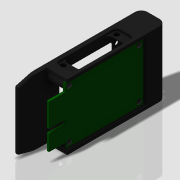
# Autodesk Inventor part: HighSpeedIOShield01
Saved by Autodesk Inventor 2013 (Build 170138000, 138)
## iProperties
Created: 2014-07-14
Part Number: HighSpeedIOShield01
Material: PCB(1)
Document SubType Name: Modeling
Designer: spichelh
Density: 1 g/cm^3
Author: spichelh
Autodesk Inventor part; units mm, degrees
ref_plane "YZ Plane" through (0, 0, 0) normal (1, 0, 0) x (0, 1, 0)
ref_plane "XZ Plane" through (0, 0, 0) normal (0, 1, 0) x (-1, 0, 0)
ref_plane "XY Plane" through (0, 0, 0) normal (0, 0, 1) x (1, 0, 0)
sketch "Sketch1" plane through (0, 0, 0) normal (1, 0, 0) x (0, 1, 0)
  line L0 (0, 0) -> (27.94, 0)
  line L1 (27.94, 0) -> (27.94, 38.1)
  line L2 (13.97, 0) -> (13.97, 11.6982) construction
  circle A0 centre (2, 2) radius 1.25
  circle A1 centre (25.94, 2) radius 1.25
  line L3 (0, 38.1) -> (2.74, 38.1)
  line L4 (2.74, 38.1) -> (2.74, 46)
  line L5 (2.74, 46) -> (10.54, 46)
  line L6 (10.54, 46) -> (10.54, 38.1)
  line L7 (10.54, 38.1) -> (12.54, 38.1)
  line L8 (12.54, 38.1) -> (12.54, 46)
  line L9 (12.54, 46) -> (24.04, 46)
  line L10 (24.04, 46) -> (24.04, 38.1)
  line L11 (24.04, 38.1) -> (27.94, 38.1)
  line L12 (0, 0) -> (0, 38.1)
  circle A2 centre (2, 36.1) radius 1.25
  circle A3 centre (25.94, 36.1) radius 1.25
  point P0 (13.97, 5.8491)
  dimension "d0" = 27.94
  dimension "d5" = 2.5
  dimension "d6" = 2
  dimension "d21" = 7.8
  dimension "d23" = 2
  dimension "d24" = 11.5
  dimension "d27" = 38.1
  dimension "d29" = 3.9
  dimension "d30" = 7.9
  dimension "d31" = 2
  dimension "d32" = 2.5
  dimension "d33" = 2
  dimension "d34" = 2
  constraints: 27 end point, 4 centre point, 3 collinear, 2 midpoint, 2 perpendicular, 2 symmetric about line, 2 vertical, 1 horizontal, 1 parallel, 2 other
  measures "d0" distance of L0.start L0.end
  measures "d5" diameter of A0
  measures "d6" distance from line of L0 A0.centre
  measures "d21" distance between parallel lines of L6 L4
  measures "d23" distance between parallel lines of L6 L8
  measures "d24" distance between parallel lines of L8 L10
  measures "d27" distance of L1.end L0.end
  measures "d29" distance between parallel lines of L10 L1
  measures "d30" distance between parallel lines of L3 L5
  measures "d31" distance from line of L12 A0.centre
  measures "d32" diameter of A2
  measures "d33" distance from line of L12 A2.centre
  measures "d34" distance from line of L3 A2.centre
extrude "Extrusion1" add sketch "Sketch1" along normal blind 1
sketch "Sketch2" plane through (0, 0, 0) normal (-1, 0, 0) x (0, 0, 1)
  circle A0 centre (2, 25.94) radius 1.25 projected
  circle A1 centre (2, 2) radius 1.25 projected
  circle A2 centre (36.1, 25.94) radius 1.25 projected
  circle A3 centre (36.1, 2) radius 1.25 projected
  circle A4 centre (36.1, 2) radius 2
  circle A5 centre (36.1, 25.94) radius 2
  circle A6 centre (2, 25.94) radius 2
  circle A7 centre (2, 2) radius 2
  dimension "d35" = 4
  dimension "d38" = 4
  dimension "d39" = 4
  dimension "d40" = 4
  constraints: 4 centre point, 4 coincident
  measures "d35" diameter of A4
  measures "d38" diameter of A5
  measures "d39" diameter of A6
  measures "d40" diameter of A7
extrude "Extrusion2" add sketch "Sketch2" along normal blind 8
sketch "Sketch3" plane through (-8, 25.94, 2) normal (-1, 0, 0) x (0, 0, 1)
  line L0 (44, -1.9) -> (44, -13.4) projected
  line L1 (44, 4) -> (50, 2.3923)
  line L2 (50, 2.3923) -> (50, -26.3323)
  line L3 (50, -26.3323) -> (45.0725, -27.6526)
  line L4 (45.0725, -27.6526) -> (44, -27.94)
  line L5 (44, -27.94) -> (-4, -27.94)
  line L6 (-4, -27.94) -> (-4, 4)
  line L7 (-4, 4) -> (44, 4)
  line L8 (-2, -25.94) -> (-2, 2) projected
  line L9 (-2, 2) -> (36.1, 2) projected
  line L10 (36.1, -25.94) -> (-2, -25.94) projected
  dimension "d43" = 105
  dimension "d44" = 105
  dimension "d45" = 2
  dimension "d46" = 2
  dimension "d47" = 2
  dimension "d48" = 6
  constraints: 14 end point, 3 perpendicular, 2 point on line, 1 collinear, 1 parallel
  measures "d43" angle of L1 L2
  measures "d44" angle of L3 L2
  measures "d45" distance between parallel lines of L6 L8
  measures "d46" distance between parallel lines of L7 L9
  measures "d47" distance between parallel lines of L5 L10
  measures "d48" distance between parallel lines of L0 L2
extrude "Extrusion3" add sketch "Sketch3" along normal blind 2
sketch "Sketch4" plane through (-8, 25.94, 2) normal (1, 0, 0) x (0, 0, -1)
  line L0 (-44, -27.94) -> (4, -27.94) projected
  line L1 (4, -27.94) -> (4, 4) projected
  line L2 (4, 4) -> (-44, 4) projected
  line L3 (2.5, 2.5) -> (2.5, -26.44)
  line L4 (2.5, -26.44) -> (-36.1, -26.44)
  line L5 (-36.1, 2) -> (-36.1, -1.9) projected
  line L6 (-36.1, 2.5) -> (-36.1, 4)
  line L7 (-36.1, -26.44) -> (-36.1, -27.94)
  line L8 (-36.1, 2.5) -> (2.5, 2.5)
  point P0 (2, -25.94)
  dimension "d51" = 1.5
  dimension "d52" = 1.5
  dimension "d53" = 1.5
  constraints: 10 end point, 2 collinear, 2 perpendicular, 2 point on line
  measures "d51" distance between parallel lines of L3 L1
  measures "d52" distance between parallel lines of L2 L8
  measures "d53" distance between parallel lines of L0 L4
extrude "Extrusion4" add sketch "Sketch4" along normal blind 10
fillet "Fillet1" radius 1 4 edges at (-3, 28.44, -0.5) (-3, -0.5, -0.5) (-9, 28.3323, 52) (-9, -0.3923, 52)
fillet "Fillet2" radius 1 10 edges at (-8, -0.2337, 51.7934) (-8, -1.2955, 48.6294) (-8, 28.1737, 51.7934) (-8, 29.2355, 48.6294) (-8, 13.97, 52) (-10, 13.97, 52) (-10, -0.2337, 51.7934) (-10, -1.2955, 48.6294) (-10, 29.2355, 48.6294) (-10, 28.1737, 51.7934)
thread "Thread1" size "M3x0.5" class "6H" standard "ANSI Metric M Profile" full length
thread "Thread2" size "M3x0.5" class "6H" standard "ANSI Metric M Profile" full length
thread "Thread3" size "M3x0.5" class "6H" standard "ANSI Metric M Profile" full length
thread "Thread4" size "M3x0.5" class "6H" standard "ANSI Metric M Profile" full length
sketch "Sketch6" plane through (2, -2, -2) normal (0, 0, -1) x (-1, 0, 0)
  line L0 (8.5, 30.44) -> (3.5, 30.44)
  line L1 (1.5, 28.44) -> (1.5, 3.5)
  line L2 (3.5, 1.5) -> (8.5, 1.5)
  line L3 (10.5, 3.5) -> (10.5, 28.44)
  arc A0 (3.5, 30.44) -> (1.5, 28.44) centre (3.5, 28.44) ccw
  arc A1 (10.5, 28.44) -> (8.5, 30.44) centre (8.5, 28.44) ccw
  arc A2 (8.5, 1.5) -> (10.5, 3.5) centre (8.5, 3.5) ccw
  arc A3 (1.5, 3.5) -> (3.5, 1.5) centre (3.5, 3.5) ccw
  line L4 (12, 31.94) -> (0, 31.94) projected
  line L5 (12, 31.94) -> (12, 0) projected
  line L6 (12, 0) -> (0, 0) projected
  line L7 (0, 0) -> (0, 31.94) projected
  dimension "d106" = 2
  dimension "d107" = 1.5
  dimension "d108" = 1.5
  dimension "d109" = 1.5
  dimension "d110" = 1.5
  constraints: 8 end point, 8 point on circle, 8 tangent, 4 centre point, 3 equal radius, 2 parallel, 1 horizontal, 1 perpendicular
  measures "d106" radius of A0
  measures "d107" distance between parallel lines of L4 L0
  measures "d108" distance between parallel lines of L3 L5
  measures "d109" distance between parallel lines of L6 L2
  measures "d110" distance between parallel lines of L7 L1
extrude "Extrusion6" cut sketch "Sketch6" against normal blind 0.1 contours A1 L3 A2 L2 A3 L1 A0 L0
sketch "Sketch7" plane through (-10, 25.94, 2) normal (-1, 0, 0) x (0, 0, 1)
  line L0 (40.1363, 4) -> (-4, 4) projected
  line L1 (1.46, -1) -> (32, -1)
  line L2 (34, -3) -> (34, -20.94)
  line L3 (32, -22.94) -> (1.46, -22.94)
  line L4 (-0.54, -20.94) -> (-0.54, -3)
  arc A0 (34, -3) -> (32, -1) centre (32, -3) ccw
  arc A1 (1.46, -1) -> (-0.54, -3) centre (1.46, -3) ccw
  arc A2 (-0.54, -20.94) -> (1.46, -22.94) centre (1.46, -20.94) ccw
  arc A3 (32, -22.94) -> (34, -20.94) centre (32, -20.94) ccw
  line L5 (-4.54, 4) -> (-4.54, -27.94) projected
  line L6 (-4, -27.94) -> (40.1363, -27.94) projected
  line L7 (49, 1.625) -> (49, -25.565) projected
  point P0 (-3.54, 4.54)
  point P1 (-2, -25.94)
  point P2 (34, -22.94)
  point P3 (34, -1)
  point P4 (-0.54, -22.94)
  point P5 (-4, 4)
  dimension "d83" = 2
  dimension "d84" = 5
  dimension "d85" = 4
  dimension "d136" = 5
  dimension "d137" = 15
  constraints: 8 end point, 8 point on circle, 8 tangent, 6 point on line, 4 centre point, 3 equal radius, 2 parallel, 1 horizontal, 1 perpendicular, 1 other
  measures "d83" radius of A0
  measures "d85" distance between parallel lines of L5 L4
  measures "d136" distance between parallel lines of L6 L3
  measures "d137" distance between parallel lines of L7 L2
extrude "Extrusion7" cut sketch "Sketch7" against normal blind 1
sketch "Sketch8" plane through (-10, -2, -2) normal (0, 0, -1) x (-1, 0, 0)
  line L0 (0, 0) -> (-12, 0) projected
  line L1 (0, 31.94) -> (0, 0) projected
  line L2 (0, 31.94) -> (-12, 31.94) projected
  line L3 (-12, 0) -> (-12, 31.94) projected
  line L4 (-3.5, 1.5) -> (-8.5, 1.5)
  line L5 (-10.5, 3.5) -> (-10.5, 28.44)
  line L6 (-8.5, 30.44) -> (-3.5, 30.44)
  line L7 (-1.5, 28.44) -> (-1.5, 3.5)
  arc A0 (-3.5, 1.5) -> (-1.5, 3.5) centre (-3.5, 3.5) ccw
  arc A1 (-10.5, 3.5) -> (-8.5, 1.5) centre (-8.5, 3.5) ccw
  arc A2 (-8.5, 30.44) -> (-10.5, 28.44) centre (-8.5, 28.44) ccw
  arc A3 (-1.5, 28.44) -> (-3.5, 30.44) centre (-3.5, 28.44) ccw
  point P0 (-10, 2)
  dimension "d88" = 1.5
  dimension "d89" = 2
  constraints: 8 end point, 8 point on circle, 8 tangent, 4 centre point, 3 equal radius, 3 other
  measures "d88" distance between parallel lines of L1 L7
  measures "d89" radius of A0
extrude "Extrusion8" add sketch "Sketch8" along normal blind 8
fillet "Fillet4" radius 3 2 edges at (-10, 13.97, -10) (2, 13.97, -10)
sketch "Sketch5" plane through (-8, 29.94, 38.1) normal (0, 1, 0) x (1, 0, 0)
  line L0 (-2, -4.0363) -> (-2, 40.1) projected
  line L1 (-2, 40.1) -> (10, 40.1) projected
  line L2 (2, 34.1) -> (6.5, 34.1)
  line L3 (8.5, 32.1) -> (8.5, 6)
  line L4 (6.5, 4) -> (2, 4)
  line L5 (0, 6) -> (0, 32.1)
  arc A0 (8.5, 32.1) -> (6.5, 34.1) centre (6.5, 32.1) ccw
  arc A1 (6.5, 4) -> (8.5, 6) centre (6.5, 6) ccw
  arc A2 (0, 6) -> (2, 4) centre (2, 6) ccw
  arc A3 (2, 34.1) -> (0, 32.1) centre (2, 32.1) ccw
  line L6 (0, 0) -> (10, 0) projected
  line L7 (10, 40.1) -> (10, 0) projected
  line L8 (1, 48.1) -> (7, 48.1) projected
  point P0 (-1, 40.1)
  point P1 (-2, 39.1)
  point P2 (8, 38.1)
  point P3 (8.5, 4)
  point P4 (8.5, 34.1)
  point P5 (0, 4)
  dimension "d69" = 2
  dimension "d70" = 2
  dimension "d71" = 6
  dimension "d93" = 1.5
  dimension "d94" = 4
  dimension "d125" = 14
  constraints: 8 end point, 8 point on circle, 8 tangent, 6 point on line, 4 centre point, 3 equal radius, 2 parallel, 1 horizontal, 1 perpendicular
  measures "d69" radius of A0
  measures "d70" distance between parallel lines of L0 L5
  measures "d71" distance between parallel lines of L1 L2
  measures "d93" distance between parallel lines of L7 L3
  measures "d94" distance between parallel lines of L6 L4
  measures "d125" distance between parallel lines of L8 L2
extrude "Extrusion5" cut sketch "Sketch5" against normal blind 1
sketch "Sketch9" plane through (-8, 28.94, 38.1) normal (0, 1, 0) x (1, 0, 0)
  line L0 (2, 34.1) -> (6.5, 34.1) projected
  line L1 (0, 6) -> (0, 32.1) projected
  line L2 (6.5, 4) -> (2, 4) projected
  line L3 (8.5, 32.1) -> (8.5, 6) projected
  line L4 (2, 30.1) -> (6.5, 30.1)
  line L5 (8.5, 28.1) -> (8.5, 10)
  line L6 (6.5, 8) -> (2, 8)
  line L7 (0, 10) -> (0, 28.1)
  arc A0 (2, 30.1) -> (0, 28.1) centre (2, 28.1) ccw
  arc A1 (8.5, 28.1) -> (6.5, 30.1) centre (6.5, 28.1) ccw
  arc A2 (6.5, 8) -> (8.5, 10) centre (6.5, 10) ccw
  arc A3 (0, 10) -> (2, 8) centre (2, 10) ccw
  circle A4 centre (2, 6) radius 1.25
  circle A5 centre (2, 32.1) radius 1.25
  point P0 (8, 38.1)
  point P1 (0, 30.1)
  point P2 (8.5, 8)
  dimension "d95" = 2
  dimension "d96" = 4
  dimension "d97" = 4
  dimension "d98" = 2.5
  dimension "d99" = 2
  dimension "d100" = 2.5
  dimension "d104" = 2
  dimension "d105" = 2
  dimension "d147" = 2
  constraints: 8 end point, 8 point on circle, 8 tangent, 6 centre point, 6 point on line, 3 equal radius, 2 parallel, 1 horizontal, 1 perpendicular
  measures "d95" radius of A0
  measures "d96" distance between parallel lines of L6 L2
  measures "d97" distance between parallel lines of L0 L4
  measures "d98" diameter of A4
  measures "d99" distance from line of A4.centre L2
  measures "d100" diameter of A5
  measures "d104" distance from line of L1 A5.centre
  measures "d105" distance from line of L1 A4.centre
  measures "d147" distance from line of L4 A5.centre
extrude "Extrusion9" cut sketch "Sketch9" against normal blind 1
sketch "Sketch10" plane through (2, -2, -1.9) normal (0, 0, -1) x (-1, 0, 0)
  line L0 (1.5, 3.5) -> (1.5, 28.44) projected
  line L1 (8.5, 1.5) -> (3.5, 1.5) projected
  line L2 (10.5, 28.44) -> (10.5, 3.5) projected
  line L3 (3.5, 30.44) -> (8.5, 30.44) projected
  line L4 (3.5, 26.44) -> (8.5, 26.44)
  line L5 (10.5, 24.44) -> (10.5, 7.5)
  line L6 (8.5, 5.5) -> (3.5, 5.5)
  line L7 (1.5, 7.5) -> (1.5, 24.44)
  arc A0 (3.5, 26.44) -> (1.5, 24.44) centre (3.5, 24.44) ccw
  arc A1 (10.5, 24.44) -> (8.5, 26.44) centre (8.5, 24.44) ccw
  arc A2 (8.5, 5.5) -> (10.5, 7.5) centre (8.5, 7.5) ccw
  arc A3 (1.5, 7.5) -> (3.5, 5.5) centre (3.5, 7.5) ccw
  arc A4 (8.5, 1.5) -> (10.5, 3.5) centre (8.5, 3.5) ccw projected
  circle A5 centre (3.5, 28.44) radius 1.25
  circle A6 centre (8.5, 3.5) radius 1.25
  point P0 (2, 2)
  point P1 (1.5, 26.44)
  point P2 (10.5, 5.5)
  dimension "d111" = 2
  dimension "d112" = 4
  dimension "d113" = 4
  dimension "d116" = 2.5
  dimension "d117" = 2
  dimension "d118" = 2
  dimension "d119" = 2.5
  constraints: 8 end point, 8 point on circle, 8 tangent, 6 centre point, 6 point on line, 3 equal radius, 2 parallel, 1 coincident, 1 horizontal, 1 perpendicular
  measures "d111" radius of A0
  measures "d112" distance between parallel lines of L4 L3
  measures "d113" distance between parallel lines of L1 L6
  measures "d116" diameter of A5
  measures "d117" distance from line of L3 A5.centre
  measures "d118" distance from line of L0 A5.centre
  measures "d119" diameter of A6
extrude "Extrusion10" cut sketch "Sketch10" against normal blind 1.9
sketch "Sketch11" plane through (-8, -2, 38.1) normal (0, -1, 0) x (1, 0, 0)
  line L0 (10, 0) -> (10, -45.1) projected
  line L1 (0, 0) -> (10, 0) projected
  line L2 (-2, 4.0363) -> (-2, -45.1) projected
  line L3 (7, -48.1) -> (1, -48.1) projected
  line L4 (2, -4) -> (6.5, -4)
  line L5 (8.5, -6) -> (8.5, -32.1)
  line L6 (6.5, -34.1) -> (2, -34.1)
  line L7 (0, -32.1) -> (0, -6)
  arc A0 (2, -4) -> (0, -6) centre (2, -6) ccw
  arc A1 (8.5, -6) -> (6.5, -4) centre (6.5, -6) ccw
  arc A2 (6.5, -34.1) -> (8.5, -32.1) centre (6.5, -32.1) ccw
  arc A3 (0, -32.1) -> (2, -34.1) centre (2, -32.1) ccw
  point P0 (8, -38.1)
  dimension "d120" = 2
  dimension "d121" = 4
  dimension "d122" = 14
  dimension "d123" = 1.5
  dimension "d124" = 2
  constraints: 8 end point, 8 point on circle, 8 tangent, 4 centre point, 3 equal radius, 2 parallel, 1 horizontal, 1 perpendicular
  measures "d120" radius of A0
  measures "d121" distance between parallel lines of L1 L4
  measures "d122" distance between parallel lines of L3 L6
  measures "d123" distance between parallel lines of L5 L0
  measures "d124" distance between parallel lines of L2 L7
extrude "Extrusion11" cut sketch "Sketch11" against normal blind 1
sketch "Sketch12" plane through (-8, -1, 38.1) normal (0, -1, 0) x (1, 0, 0)
  line L0 (2, -4) -> (6.5, -4) projected
  arc A0 (2, -4) -> (0, -6) centre (2, -6) ccw projected
  line L1 (0, -32.1) -> (0, -6) projected
  line L2 (6.5, -34.1) -> (2, -34.1) projected
  line L3 (8.5, -6) -> (8.5, -32.1) projected
  line L4 (2, -8) -> (6.5, -8)
  line L5 (8.5, -10) -> (8.5, -28.1)
  line L6 (6.5, -30.1) -> (2, -30.1)
  line L7 (0, -28.1) -> (0, -10)
  arc A1 (8.5, -10) -> (6.5, -8) centre (6.5, -10) ccw
  arc A2 (6.5, -30.1) -> (8.5, -28.1) centre (6.5, -28.1) ccw
  arc A3 (0, -28.1) -> (2, -30.1) centre (2, -28.1) ccw
  arc A4 (2, -8) -> (0, -10) centre (2, -10) ccw
  circle A5 centre (2, -6) radius 1.25
  arc A6 (0, -32.1) -> (2, -34.1) centre (2, -32.1) ccw projected
  circle A7 centre (2, -32.1) radius 1.25
  point P0 (8, -38.1)
  point P1 (0, -8)
  point P2 (8.5, -30.1)
  dimension "d128" = 2
  dimension "d129" = 4
  dimension "d130" = 4
  dimension "d131" = 2.5
  dimension "d135" = 2.5
  constraints: 8 end point, 8 point on circle, 8 tangent, 6 centre point, 6 point on line, 3 equal radius, 2 coincident, 2 parallel, 1 horizontal, 1 perpendicular
  measures "d128" radius of A1
  measures "d129" distance between parallel lines of L0 L4
  measures "d130" distance between parallel lines of L6 L2
  measures "d131" diameter of A5
  measures "d135" diameter of A7
extrude "Extrusion12" cut sketch "Sketch12" against normal blind 1
sketch "Sketch13" plane through (-9, 25.94, 2) normal (-1, 0, 0) x (0, 0, 1)
  line L0 (1.46, -1) -> (32, -1) projected
  arc A0 (1.46, -1) -> (-0.54, -3) centre (1.46, -3) ccw projected
  line L1 (-0.54, -20.94) -> (-0.54, -3) projected
  arc A1 (-0.54, -20.94) -> (1.46, -22.94) centre (1.46, -20.94) ccw projected
  line L2 (32, -22.94) -> (1.46, -22.94) projected
  arc A2 (32, -22.94) -> (34, -20.94) centre (32, -20.94) ccw projected
  line L3 (34, -3) -> (34, -20.94) projected
  arc A3 (34, -3) -> (32, -1) centre (32, -3) ccw projected
  line L4 (5.46, -1) -> (28, -1)
  line L5 (30, -3) -> (30, -20.94)
  line L6 (28, -22.94) -> (5.46, -22.94)
  line L7 (3.46, -20.94) -> (3.46, -3)
  arc A4 (5.46, -1) -> (3.46, -3) centre (5.46, -3) ccw
  arc A5 (3.46, -20.94) -> (5.46, -22.94) centre (5.46, -20.94) ccw
  arc A6 (28, -22.94) -> (30, -20.94) centre (28, -20.94) ccw
  arc A7 (30, -3) -> (28, -1) centre (28, -3) ccw
  circle A8 centre (1.46, -3) radius 1.25
  circle A9 centre (32, -20.94) radius 1.25
  circle A10 centre (32, -3) radius 1.25
  circle A11 centre (1.46, -20.94) radius 1.25
  point P0 (-2, -25.94)
  point P1 (3.46, -1)
  point P2 (30, -22.94)
  dimension "d138" = 2
  dimension "d139" = 4
  dimension "d140" = 4
  dimension "d141" = 2.5
  dimension "d142" = 2.5
  dimension "d143" = 2.5
  dimension "d144" = 2.5
  constraints: 8 centre point, 8 end point, 8 point on circle, 8 tangent, 6 point on line, 4 coincident, 3 equal radius, 2 parallel, 1 horizontal, 1 perpendicular
  measures "d138" radius of A4
  measures "d139" distance between parallel lines of L1 L7
  measures "d140" distance between parallel lines of L3 L5
  measures "d141" diameter of A8
  measures "d142" diameter of A9
  measures "d143" diameter of A10
  measures "d144" diameter of A11
extrude "Extrusion13" cut sketch "Sketch13" against normal blind 1 contours L0 A7 L5 A6 L2 A5 L7 A4 | A8 | A9 | A10 | A11
body "Solid1"
